Autodesk Inventor part; units mm, degrees
(part 3 of 15)
  line L366 (-4.016, 12.192) -> (-4.016, 13.208)
  arc A1008 (-3.9652, 13.208) -> (-4.0668, 13.208) centre (-4.016, 13.208) ccw
  arc A1009 (-4.0668, 12.192) -> (-3.9652, 12.192) centre (-4.016, 12.192) ccw
  arc A1010 (39.084, 48.5588) -> (39.084, 48.4572) centre (39.084, 48.508) ccw
  line L367 (-17.016, 17.208) -> (-14.984, 17.208)
  arc A1011 (-14.984, 17.1572) -> (-14.984, 17.2588) centre (-14.984, 17.208) ccw
  arc A1012 (-17.016, 17.2588) -> (-17.016, 17.1572) centre (-17.016, 17.208) ccw
  line L368 (-14.984, 17.208) -> (-14.984, 16.192)
  arc A1013 (-15.0348, 16.192) -> (-14.9332, 16.192) centre (-14.984, 16.192) ccw
  arc A1014 (-14.9332, 17.208) -> (-15.0348, 17.208) centre (-14.984, 17.208) ccw
  line L369 (-14.984, 16.192) -> (-17.016, 16.192)
  arc A1015 (-17.016, 16.2428) -> (-17.016, 16.1412) centre (-17.016, 16.192) ccw
  arc A1016 (-14.984, 16.1412) -> (-14.984, 16.2428) centre (-14.984, 16.192) ccw
  line L370 (-17.016, 16.192) -> (-17.016, 17.208)
  arc A1017 (-16.9652, 17.208) -> (-17.0668, 17.208) centre (-17.016, 17.208) ccw
  arc A1018 (-17.0668, 16.192) -> (-16.9652, 16.192) centre (-17.016, 16.192) ccw
  line L371 (41.116, 48.508) -> (41.116, 47.492)
  line L372 (-16.984, 0.192) -> (-19.016, 0.192)
  arc A1019 (-19.016, 0.2428) -> (-19.016, 0.1412) centre (-19.016, 0.192) ccw
  arc A1020 (-16.984, 0.1412) -> (-16.984, 0.2428) centre (-16.984, 0.192) ccw
  line L373 (-19.016, 0.192) -> (-19.016, 1.208)
  arc A1021 (-18.9652, 1.208) -> (-19.0668, 1.208) centre (-19.016, 1.208) ccw
  arc A1022 (-19.0668, 0.192) -> (-18.9652, 0.192) centre (-19.016, 0.192) ccw
  line L374 (-19.016, 1.208) -> (-16.984, 1.208)
  arc A1023 (-16.984, 1.1572) -> (-16.984, 1.2588) centre (-16.984, 1.208) ccw
  arc A1024 (-19.016, 1.2588) -> (-19.016, 1.1572) centre (-19.016, 1.208) ccw
  line L375 (-16.984, 1.208) -> (-16.984, 0.192)
  arc A1025 (-17.0348, 0.192) -> (-16.9332, 0.192) centre (-16.984, 0.192) ccw
  arc A1026 (-16.9332, 1.208) -> (-17.0348, 1.208) centre (-16.984, 1.208) ccw
  arc A1027 (41.0652, 47.492) -> (41.1668, 47.492) centre (41.116, 47.492) ccw
  line L376 (7.008, 13.216) -> (7.008, 11.184)
  arc A1028 (6.9572, 11.184) -> (7.0588, 11.184) centre (7.008, 11.184) ccw
  arc A1029 (7.0588, 13.216) -> (6.9572, 13.216) centre (7.008, 13.216) ccw
  line L377 (7.008, 11.184) -> (5.992, 11.184)
  arc A1030 (5.992, 11.2348) -> (5.992, 11.1332) centre (5.992, 11.184) ccw
  arc A1031 (7.008, 11.1332) -> (7.008, 11.2348) centre (7.008, 11.184) ccw
  line L378 (5.992, 11.184) -> (5.992, 13.216)
  arc A1032 (6.0428, 13.216) -> (5.9412, 13.216) centre (5.992, 13.216) ccw
  arc A1033 (5.9412, 11.184) -> (6.0428, 11.184) centre (5.992, 11.184) ccw
  line L379 (5.992, 13.216) -> (7.008, 13.216)
  arc A1034 (7.008, 13.1652) -> (7.008, 13.2668) centre (7.008, 13.216) ccw
  arc A1035 (5.992, 13.2668) -> (5.992, 13.1652) centre (5.992, 13.216) ccw
  arc A1036 (41.1668, 48.508) -> (41.0652, 48.508) centre (41.116, 48.508) ccw
  line L380 (-15.984, 6.192) -> (-18.016, 6.192)
  arc A1037 (-18.016, 6.2428) -> (-18.016, 6.1412) centre (-18.016, 6.192) ccw
  arc A1038 (-15.984, 6.1412) -> (-15.984, 6.2428) centre (-15.984, 6.192) ccw
  line L381 (-18.016, 6.192) -> (-18.016, 7.208)
  arc A1039 (-17.9652, 7.208) -> (-18.0668, 7.208) centre (-18.016, 7.208) ccw
  arc A1040 (-18.0668, 6.192) -> (-17.9652, 6.192) centre (-18.016, 6.192) ccw
  line L382 (-18.016, 7.208) -> (-15.984, 7.208)
  arc A1041 (-15.984, 7.1572) -> (-15.984, 7.2588) centre (-15.984, 7.208) ccw
  arc A1042 (-18.016, 7.2588) -> (-18.016, 7.1572) centre (-18.016, 7.208) ccw
  line L383 (-15.984, 7.208) -> (-15.984, 6.192)
  arc A1043 (-16.0348, 6.192) -> (-15.9332, 6.192) centre (-15.984, 6.192) ccw
  arc A1044 (-15.9332, 7.208) -> (-16.0348, 7.208) centre (-15.984, 7.208) ccw
  line L384 (41.116, 48.492) -> (39.084, 48.492)
  line L385 (-1.984, 11.192) -> (-4.016, 11.192)
  arc A1045 (-4.016, 11.2428) -> (-4.016, 11.1412) centre (-4.016, 11.192) ccw
  arc A1046 (-1.984, 11.1412) -> (-1.984, 11.2428) centre (-1.984, 11.192) ccw
  line L386 (-4.016, 11.192) -> (-4.016, 12.208)
  arc A1047 (-3.9652, 12.208) -> (-4.0668, 12.208) centre (-4.016, 12.208) ccw
  arc A1048 (-4.0668, 11.192) -> (-3.9652, 11.192) centre (-4.016, 11.192) ccw
  line L387 (-4.016, 12.208) -> (-1.984, 12.208)
  arc A1049 (-1.984, 12.1572) -> (-1.984, 12.2588) centre (-1.984, 12.208) ccw
  arc A1050 (-4.016, 12.2588) -> (-4.016, 12.1572) centre (-4.016, 12.208) ccw
  line L388 (-1.984, 12.208) -> (-1.984, 11.192)
  arc A1051 (-2.0348, 11.192) -> (-1.9332, 11.192) centre (-1.984, 11.192) ccw
  arc A1052 (-1.9332, 12.208) -> (-2.0348, 12.208) centre (-1.984, 12.208) ccw
  arc A1053 (39.084, 48.5428) -> (39.084, 48.4412) centre (39.084, 48.492) ccw
  line L389 (-17.984, 17.192) -> (-20.016, 17.192)
  arc A1054 (-20.016, 17.2428) -> (-20.016, 17.1412) centre (-20.016, 17.192) ccw
  arc A1055 (-17.984, 17.1412) -> (-17.984, 17.2428) centre (-17.984, 17.192) ccw
  line L390 (-20.016, 17.192) -> (-20.016, 18.208)
  arc A1056 (-19.9652, 18.208) -> (-20.0668, 18.208) centre (-20.016, 18.208) ccw
  arc A1057 (-20.0668, 17.192) -> (-19.9652, 17.192) centre (-20.016, 17.192) ccw
  line L391 (-20.016, 18.208) -> (-17.984, 18.208)
  arc A1058 (-17.984, 18.1572) -> (-17.984, 18.2588) centre (-17.984, 18.208) ccw
  arc A1059 (-20.016, 18.2588) -> (-20.016, 18.1572) centre (-20.016, 18.208) ccw
  line L392 (-17.984, 18.208) -> (-17.984, 17.192)
  arc A1060 (-18.0348, 17.192) -> (-17.9332, 17.192) centre (-17.984, 17.192) ccw
  arc A1061 (-17.9332, 18.208) -> (-18.0348, 18.208) centre (-17.984, 18.208) ccw
  arc A1062 (41.116, 48.4412) -> (41.116, 48.5428) centre (41.116, 48.492) ccw
  line L393 (-18.008, 12.184) -> (-18.008, 14.216)
  arc A1063 (-17.9572, 14.216) -> (-18.0588, 14.216) centre (-18.008, 14.216) ccw
  arc A1064 (-18.0588, 12.184) -> (-17.9572, 12.184) centre (-18.008, 12.184) ccw
  line L394 (-18.008, 14.216) -> (-16.992, 14.216)
  arc A1065 (-16.992, 14.1652) -> (-16.992, 14.2668) centre (-16.992, 14.216) ccw
  arc A1066 (-18.008, 14.2668) -> (-18.008, 14.1652) centre (-18.008, 14.216) ccw
  line L395 (-16.992, 14.216) -> (-16.992, 12.184)
  arc A1067 (-17.0428, 12.184) -> (-16.9412, 12.184) centre (-16.992, 12.184) ccw
  arc A1068 (-16.9412, 14.216) -> (-17.0428, 14.216) centre (-16.992, 14.216) ccw
  line L396 (-16.992, 12.184) -> (-18.008, 12.184)
  arc A1069 (-18.008, 12.2348) -> (-18.008, 12.1332) centre (-18.008, 12.184) ccw
  arc A1070 (-16.992, 12.1332) -> (-16.992, 12.2348) centre (-16.992, 12.184) ccw
  line L397 (39.084, 48.492) -> (39.084, 49.508)
  line L398 (-14.992, 10.216) -> (-14.992, 8.184)
  arc A1071 (-15.0428, 8.184) -> (-14.9412, 8.184) centre (-14.992, 8.184) ccw
  arc A1072 (-14.9412, 10.216) -> (-15.0428, 10.216) centre (-14.992, 10.216) ccw
  line L399 (-14.992, 8.184) -> (-16.008, 8.184)
  arc A1073 (-16.008, 8.2348) -> (-16.008, 8.1332) centre (-16.008, 8.184) ccw
  arc A1074 (-14.992, 8.1332) -> (-14.992, 8.2348) centre (-14.992, 8.184) ccw
  line L400 (-16.008, 8.184) -> (-16.008, 10.216)
  arc A1075 (-15.9572, 10.216) -> (-16.0588, 10.216) centre (-16.008, 10.216) ccw
  arc A1076 (-16.0588, 8.184) -> (-15.9572, 8.184) centre (-16.008, 8.184) ccw
  line L401 (-16.008, 10.216) -> (-14.992, 10.216)
  arc A1077 (-14.992, 10.1652) -> (-14.992, 10.2668) centre (-14.992, 10.216) ccw
  arc A1078 (-16.008, 10.2668) -> (-16.008, 10.1652) centre (-16.008, 10.216) ccw
  arc A1079 (39.1348, 49.508) -> (39.0332, 49.508) centre (39.084, 49.508) ccw
  line L402 (3.103, 14.835) -> (5.897, 14.835)
  arc A1080 (5.897, 14.7842) -> (5.897, 14.8858) centre (5.897, 14.835) ccw
  arc A1081 (3.103, 14.8858) -> (3.103, 14.7842) centre (3.103, 14.835) ccw
  line L403 (5.897, 14.835) -> (5.897, 13.565)
  arc A1082 (5.8462, 13.565) -> (5.9478, 13.565) centre (5.897, 13.565) ccw
  arc A1083 (5.9478, 14.835) -> (5.8462, 14.835) centre (5.897, 14.835) ccw
  line L404 (5.897, 13.565) -> (3.103, 13.565)
  arc A1084 (3.103, 13.6158) -> (3.103, 13.5142) centre (3.103, 13.565) ccw
  arc A1085 (5.897, 13.5142) -> (5.897, 13.6158) centre (5.897, 13.565) ccw
  line L405 (3.103, 13.565) -> (3.103, 14.835)
  arc A1086 (3.1538, 14.835) -> (3.0522, 14.835) centre (3.103, 14.835) ccw
  arc A1087 (3.0522, 13.565) -> (3.1538, 13.565) centre (3.103, 13.565) ccw
  arc A1088 (39.0332, 48.492) -> (39.1348, 48.492) centre (39.084, 48.492) ccw
  line L406 (-3.008, 7.184) -> (-3.008, 9.216)
  arc A1089 (-2.9572, 9.216) -> (-3.0588, 9.216) centre (-3.008, 9.216) ccw
  arc A1090 (-3.0588, 7.184) -> (-2.9572, 7.184) centre (-3.008, 7.184) ccw
  line L407 (-3.008, 9.216) -> (-1.992, 9.216)
  arc A1091 (-1.992, 9.1652) -> (-1.992, 9.2668) centre (-1.992, 9.216) ccw
  arc A1092 (-3.008, 9.2668) -> (-3.008, 9.1652) centre (-3.008, 9.216) ccw
  line L408 (-1.992, 9.216) -> (-1.992, 7.184)
  arc A1093 (-2.0428, 7.184) -> (-1.9412, 7.184) centre (-1.992, 7.184) ccw
  arc A1094 (-1.9412, 9.216) -> (-2.0428, 9.216) centre (-1.992, 9.216) ccw
  line L409 (-1.992, 7.184) -> (-3.008, 7.184)
  arc A1095 (-3.008, 7.2348) -> (-3.008, 7.1332) centre (-3.008, 7.184) ccw
  arc A1096 (-1.992, 7.1332) -> (-1.992, 7.2348) centre (-1.992, 7.184) ccw
  line L410 (39.084, 49.508) -> (41.116, 49.508)
  line L411 (-15.984, 4.192) -> (-18.016, 4.192)
  arc A1097 (-18.016, 4.2428) -> (-18.016, 4.1412) centre (-18.016, 4.192) ccw
  arc A1098 (-15.984, 4.1412) -> (-15.984, 4.2428) centre (-15.984, 4.192) ccw
  line L412 (-18.016, 4.192) -> (-18.016, 5.208)
  arc A1099 (-17.9652, 5.208) -> (-18.0668, 5.208) centre (-18.016, 5.208) ccw
  arc A1100 (-18.0668, 4.192) -> (-17.9652, 4.192) centre (-18.016, 4.192) ccw
  line L413 (-18.016, 5.208) -> (-15.984, 5.208)
  arc A1101 (-15.984, 5.1572) -> (-15.984, 5.2588) centre (-15.984, 5.208) ccw
  arc A1102 (-18.016, 5.2588) -> (-18.016, 5.1572) centre (-18.016, 5.208) ccw
  line L414 (-15.984, 5.208) -> (-15.984, 4.192)
  arc A1103 (-16.0348, 4.192) -> (-15.9332, 4.192) centre (-15.984, 4.192) ccw
  arc A1104 (-15.9332, 5.208) -> (-16.0348, 5.208) centre (-15.984, 5.208) ccw
  arc A1105 (41.116, 49.4572) -> (41.116, 49.5588) centre (41.116, 49.508) ccw
  line L415 (-12.397, 4.835) -> (-9.603, 4.835)
  arc A1106 (-9.603, 4.7842) -> (-9.603, 4.8858) centre (-9.603, 4.835) ccw
  arc A1107 (-12.397, 4.8858) -> (-12.397, 4.7842) centre (-12.397, 4.835) ccw
  line L416 (-9.603, 4.835) -> (-9.603, 3.565)
  arc A1108 (-9.6538, 3.565) -> (-9.5522, 3.565) centre (-9.603, 3.565) ccw
  arc A1109 (-9.5522, 4.835) -> (-9.6538, 4.835) centre (-9.603, 4.835) ccw
  line L417 (-9.603, 3.565) -> (-12.397, 3.565)
  arc A1110 (-12.397, 3.6158) -> (-12.397, 3.5142) centre (-12.397, 3.565) ccw
  arc A1111 (-9.603, 3.5142) -> (-9.603, 3.6158) centre (-9.603, 3.565) ccw
  line L418 (-12.397, 3.565) -> (-12.397, 4.835)
  arc A1112 (-12.3462, 4.835) -> (-12.4478, 4.835) centre (-12.397, 4.835) ccw
  arc A1113 (-12.4478, 3.565) -> (-12.3462, 3.565) centre (-12.397, 3.565) ccw
  arc A1114 (39.084, 49.5588) -> (39.084, 49.4572) centre (39.084, 49.508) ccw
  line L419 (-6.165, 16.097) -> (-6.165, 13.303)
  arc A1115 (-6.2158, 13.303) -> (-6.1142, 13.303) centre (-6.165, 13.303) ccw
  arc A1116 (-6.1142, 16.097) -> (-6.2158, 16.097) centre (-6.165, 16.097) ccw
  line L420 (-6.165, 13.303) -> (-7.435, 13.303)
  arc A1117 (-7.435, 13.3538) -> (-7.435, 13.2522) centre (-7.435, 13.303) ccw
  arc A1118 (-6.165, 13.2522) -> (-6.165, 13.3538) centre (-6.165, 13.303) ccw
  line L421 (-7.435, 13.303) -> (-7.435, 16.097)
  arc A1119 (-7.3842, 16.097) -> (-7.4858, 16.097) centre (-7.435, 16.097) ccw
  arc A1120 (-7.4858, 13.303) -> (-7.3842, 13.303) centre (-7.435, 13.303) ccw
  line L422 (-7.435, 16.097) -> (-6.165, 16.097)
  arc A1121 (-6.165, 16.0462) -> (-6.165, 16.1478) centre (-6.165, 16.097) ccw
  arc A1122 (-7.435, 16.1478) -> (-7.435, 16.0462) centre (-7.435, 16.097) ccw
  line L423 (41.116, 49.508) -> (41.116, 48.492)
  line L424 (-5.984, 12.192) -> (-8.016, 12.192)
  arc A1123 (-8.016, 12.2428) -> (-8.016, 12.1412) centre (-8.016, 12.192) ccw
  arc A1124 (-5.984, 12.1412) -> (-5.984, 12.2428) centre (-5.984, 12.192) ccw
  line L425 (-8.016, 12.192) -> (-8.016, 13.208)
  arc A1125 (-7.9652, 13.208) -> (-8.0668, 13.208) centre (-8.016, 13.208) ccw
  arc A1126 (-8.0668, 12.192) -> (-7.9652, 12.192) centre (-8.016, 12.192) ccw
  line L426 (-8.016, 13.208) -> (-5.984, 13.208)
  arc A1127 (-5.984, 13.1572) -> (-5.984, 13.2588) centre (-5.984, 13.208) ccw
  arc A1128 (-8.016, 13.2588) -> (-8.016, 13.1572) centre (-8.016, 13.208) ccw
  line L427 (-5.984, 13.208) -> (-5.984, 12.192)
  arc A1129 (-6.0348, 12.192) -> (-5.9332, 12.192) centre (-5.984, 12.192) ccw
  arc A1130 (-5.9332, 13.208) -> (-6.0348, 13.208) centre (-5.984, 13.208) ccw
  arc A1131 (41.0652, 48.492) -> (41.1668, 48.492) centre (41.116, 48.492) ccw
  line L428 (-9.865, 12.097) -> (-9.865, 9.303)
  arc A1132 (-9.9158, 9.303) -> (-9.8142, 9.303) centre (-9.865, 9.303) ccw
  arc A1133 (-9.8142, 12.097) -> (-9.9158, 12.097) centre (-9.865, 12.097) ccw
  line L429 (-9.865, 9.303) -> (-11.135, 9.303)
  arc A1134 (-11.135, 9.3538) -> (-11.135, 9.2522) centre (-11.135, 9.303) ccw
  arc A1135 (-9.865, 9.2522) -> (-9.865, 9.3538) centre (-9.865, 9.303) ccw
  line L430 (-11.135, 9.303) -> (-11.135, 12.097)
  arc A1136 (-11.0842, 12.097) -> (-11.1858, 12.097) centre (-11.135, 12.097) ccw
  arc A1137 (-11.1858, 9.303) -> (-11.0842, 9.303) centre (-11.135, 9.303) ccw
  line L431 (-11.135, 12.097) -> (-9.865, 12.097)
  arc A1138 (-9.865, 12.0462) -> (-9.865, 12.1478) centre (-9.865, 12.097) ccw
  arc A1139 (-11.135, 12.1478) -> (-11.135, 12.0462) centre (-11.135, 12.097) ccw
  arc A1140 (41.1668, 49.508) -> (41.0652, 49.508) centre (41.116, 49.508) ccw
  line L432 (-7.565, 16.097) -> (-7.565, 13.303)
  arc A1141 (-7.6158, 13.303) -> (-7.5142, 13.303) centre (-7.565, 13.303) ccw
  arc A1142 (-7.5142, 16.097) -> (-7.6158, 16.097) centre (-7.565, 16.097) ccw
  line L433 (-7.565, 13.303) -> (-8.835, 13.303)
  arc A1143 (-8.835, 13.3538) -> (-8.835, 13.2522) centre (-8.835, 13.303) ccw
  arc A1144 (-7.565, 13.2522) -> (-7.565, 13.3538) centre (-7.565, 13.303) ccw
  line L434 (-8.835, 13.303) -> (-8.835, 16.097)
  arc A1145 (-8.7842, 16.097) -> (-8.8858, 16.097) centre (-8.835, 16.097) ccw
  arc A1146 (-8.8858, 13.303) -> (-8.7842, 13.303) centre (-8.835, 13.303) ccw
  line L435 (-8.835, 16.097) -> (-7.565, 16.097)
  arc A1147 (-7.565, 16.0462) -> (-7.565, 16.1478) centre (-7.565, 16.097) ccw
  arc A1148 (-8.835, 16.1478) -> (-8.835, 16.0462) centre (-8.835, 16.097) ccw
  line L436 (41.116, 49.492) -> (39.084, 49.492)
  line L437 (-16.187, 8.076) -> (-21.013, 8.076)
  arc A1149 (-21.013, 8.1268) -> (-21.013, 8.0252) centre (-21.013, 8.076) ccw
  arc A1150 (-16.187, 8.0252) -> (-16.187, 8.1268) centre (-16.187, 8.076) ccw
  line L438 (-21.013, 8.076) -> (-21.013, 11.124)
  arc A1151 (-20.9622, 11.124) -> (-21.0638, 11.124) centre (-21.013, 11.124) ccw
  arc A1152 (-21.0638, 8.076) -> (-20.9622, 8.076) centre (-21.013, 8.076) ccw
  line L439 (-21.013, 11.124) -> (-16.187, 11.124)
  arc A1153 (-16.187, 11.0732) -> (-16.187, 11.1748) centre (-16.187, 11.124) ccw
  arc A1154 (-21.013, 11.1748) -> (-21.013, 11.0732) centre (-21.013, 11.124) ccw
  line L440 (-16.187, 11.124) -> (-16.187, 8.076)
  arc A1155 (-16.2378, 8.076) -> (-16.1362, 8.076) centre (-16.187, 8.076) ccw
  arc A1156 (-16.1362, 11.124) -> (-16.2378, 11.124) centre (-16.187, 11.124) ccw
  arc A1157 (39.084, 49.5428) -> (39.084, 49.4412) centre (39.084, 49.492) ccw
  line L441 (-24.8542, 11.089) -> (-21.1458, 11.089)
  arc A1158 (-21.1458, 11.0382) -> (-21.1458, 11.1398) centre (-21.1458, 11.089) ccw
  arc A1159 (-24.8542, 11.1398) -> (-24.8542, 11.0382) centre (-24.8542, 11.089) ccw
  line L442 (-21.1458, 11.089) -> (-21.1458, 9.311)
  arc A1160 (-21.1966, 9.311) -> (-21.095, 9.311) centre (-21.1458, 9.311) ccw
  arc A1161 (-21.095, 11.089) -> (-21.1966, 11.089) centre (-21.1458, 11.089) ccw
  line L443 (-21.1458, 9.311) -> (-24.8542, 9.311)
  arc A1162 (-24.8542, 9.3618) -> (-24.8542, 9.2602) centre (-24.8542, 9.311) ccw
  arc A1163 (-21.1458, 9.2602) -> (-21.1458, 9.3618) centre (-21.1458, 9.311) ccw
  line L444 (-24.8542, 9.311) -> (-24.8542, 11.089)
  arc A1164 (-24.8034, 11.089) -> (-24.905, 11.089) centre (-24.8542, 11.089) ccw
  arc A1165 (-24.905, 9.311) -> (-24.8034, 9.311) centre (-24.8542, 9.311) ccw
  arc A1166 (41.116, 49.4412) -> (41.116, 49.5428) centre (41.116, 49.492) ccw
  line L445 (-4.016, -2.792) -> (-1.984, -2.792)
  arc A1167 (-1.984, -2.8428) -> (-1.984, -2.7412) centre (-1.984, -2.792) ccw
  arc A1168 (-4.016, -2.7412) -> (-4.016, -2.8428) centre (-4.016, -2.792) ccw
  line L446 (-1.984, -2.792) -> (-1.984, -3.808)
  arc A1169 (-2.0348, -3.808) -> (-1.9332, -3.808) centre (-1.984, -3.808) ccw
  arc A1170 (-1.9332, -2.792) -> (-2.0348, -2.792) centre (-1.984, -2.792) ccw
  line L447 (-1.984, -3.808) -> (-4.016, -3.808)
  arc A1171 (-4.016, -3.7572) -> (-4.016, -3.8588) centre (-4.016, -3.808) ccw
  arc A1172 (-1.984, -3.8588) -> (-1.984, -3.7572) centre (-1.984, -3.808) ccw
  line L448 (-4.016, -3.808) -> (-4.016, -2.792)
  arc A1173 (-3.9652, -2.792) -> (-4.0668, -2.792) centre (-4.016, -2.792) ccw
  arc A1174 (-4.0668, -3.808) -> (-3.9652, -3.808) centre (-4.016, -3.808) ccw
  line L449 (39.084, 49.492) -> (39.084, 50.508)
  line L450 (-3.635, -7.697) -> (-3.635, -4.903)
  arc A1175 (-3.5842, -4.903) -> (-3.6858, -4.903) centre (-3.635, -4.903) ccw
  arc A1176 (-3.6858, -7.697) -> (-3.5842, -7.697) centre (-3.635, -7.697) ccw
  line L451 (-3.635, -4.903) -> (-2.365, -4.903)
  arc A1177 (-2.365, -4.9538) -> (-2.365, -4.8522) centre (-2.365, -4.903) ccw
  arc A1178 (-3.635, -4.8522) -> (-3.635, -4.9538) centre (-3.635, -4.903) ccw
  line L452 (-2.365, -4.903) -> (-2.365, -7.697)
  arc A1179 (-2.4158, -7.697) -> (-2.3142, -7.697) centre (-2.365, -7.697) ccw
  arc A1180 (-2.3142, -4.903) -> (-2.4158, -4.903) centre (-2.365, -4.903) ccw
  line L453 (-2.365, -7.697) -> (-3.635, -7.697)
  arc A1181 (-3.635, -7.6462) -> (-3.635, -7.7478) centre (-3.635, -7.697) ccw
  arc A1182 (-2.365, -7.7478) -> (-2.365, -7.6462) centre (-2.365, -7.697) ccw
  arc A1183 (39.1348, 50.508) -> (39.0332, 50.508) centre (39.084, 50.508) ccw
  line L454 (-13.811, 21.0542) -> (-13.811, 17.3458)
  arc A1184 (-13.8618, 17.3458) -> (-13.7602, 17.3458) centre (-13.811, 17.3458) ccw
  arc A1185 (-13.7602, 21.0542) -> (-13.8618, 21.0542) centre (-13.811, 21.0542) ccw
  line L455 (-13.811, 17.3458) -> (-15.589, 17.3458)
  arc A1186 (-15.589, 17.3966) -> (-15.589, 17.295) centre (-15.589, 17.3458) ccw
  arc A1187 (-13.811, 17.295) -> (-13.811, 17.3966) centre (-13.811, 17.3458) ccw
  line L456 (-15.589, 17.3458) -> (-15.589, 21.0542)
  arc A1188 (-15.5382, 21.0542) -> (-15.6398, 21.0542) centre (-15.589, 21.0542) ccw
  arc A1189 (-15.6398, 17.3458) -> (-15.5382, 17.3458) centre (-15.589, 17.3458) ccw
  line L457 (-15.589, 21.0542) -> (-13.811, 21.0542)
  arc A1190 (-13.811, 21.0034) -> (-13.811, 21.105) centre (-13.811, 21.0542) ccw
  arc A1191 (-15.589, 21.105) -> (-15.589, 21.0034) centre (-15.589, 21.0542) ccw
  arc A1192 (39.0332, 49.492) -> (39.1348, 49.492) centre (39.084, 49.492) ccw
  line L458 (-4.016, -1.792) -> (-1.984, -1.792)
  arc A1193 (-1.984, -1.8428) -> (-1.984, -1.7412) centre (-1.984, -1.792) ccw
  arc A1194 (-4.016, -1.7412) -> (-4.016, -1.8428) centre (-4.016, -1.792) ccw
  line L459 (-1.984, -1.792) -> (-1.984, -2.808)
  arc A1195 (-2.0348, -2.808) -> (-1.9332, -2.808) centre (-1.984, -2.808) ccw
  arc A1196 (-1.9332, -1.792) -> (-2.0348, -1.792) centre (-1.984, -1.792) ccw
  line L460 (-1.984, -2.808) -> (-4.016, -2.808)
  arc A1197 (-4.016, -2.7572) -> (-4.016, -2.8588) centre (-4.016, -2.808) ccw
  arc A1198 (-1.984, -2.8588) -> (-1.984, -2.7572) centre (-1.984, -2.808) ccw
  line L461 (-4.016, -2.808) -> (-4.016, -1.792)
  arc A1199 (-3.9652, -1.792) -> (-4.0668, -1.792) centre (-4.016, -1.792) ccw
  arc A1200 (-4.0668, -2.808) -> (-3.9652, -2.808) centre (-4.016, -2.808) ccw
  line L462 (39.084, 50.508) -> (41.116, 50.508)
  line L463 (1.016, -1.808) -> (-1.016, -1.808)
  arc A1201 (-1.016, -1.7572) -> (-1.016, -1.8588) centre (-1.016, -1.808) ccw
  arc A1202 (1.016, -1.8588) -> (1.016, -1.7572) centre (1.016, -1.808) ccw
  line L464 (-1.016, -1.808) -> (-1.016, -0.792)
  arc A1203 (-0.9652, -0.792) -> (-1.0668, -0.792) centre (-1.016, -0.792) ccw
  arc A1204 (-1.0668, -1.808) -> (-0.9652, -1.808) centre (-1.016, -1.808) ccw
  line L465 (-1.016, -0.792) -> (1.016, -0.792)
  arc A1205 (1.016, -0.8428) -> (1.016, -0.7412) centre (1.016, -0.792) ccw
  arc A1206 (-1.016, -0.7412) -> (-1.016, -0.8428) centre (-1.016, -0.792) ccw
  line L466 (1.016, -0.792) -> (1.016, -1.808)
  arc A1207 (0.9652, -1.808) -> (1.0668, -1.808) centre (1.016, -1.808) ccw
  arc A1208 (1.0668, -0.792) -> (0.9652, -0.792) centre (1.016, -0.792) ccw
  arc A1209 (41.116, 50.4572) -> (41.116, 50.5588) centre (41.116, 50.508) ccw
  line L467 (-15.611, 21.0542) -> (-15.611, 17.3458)
  arc A1210 (-15.6618, 17.3458) -> (-15.5602, 17.3458) centre (-15.611, 17.3458) ccw
  arc A1211 (-15.5602, 21.0542) -> (-15.6618, 21.0542) centre (-15.611, 21.0542) ccw
  line L468 (-15.611, 17.3458) -> (-17.389, 17.3458)
  arc A1212 (-17.389, 17.3966) -> (-17.389, 17.295) centre (-17.389, 17.3458) ccw
  arc A1213 (-15.611, 17.295) -> (-15.611, 17.3966) centre (-15.611, 17.3458) ccw
  line L469 (-17.389, 17.3458) -> (-17.389, 21.0542)
  arc A1214 (-17.3382, 21.0542) -> (-17.4398, 21.0542) centre (-17.389, 21.0542) ccw
  arc A1215 (-17.4398, 17.3458) -> (-17.3382, 17.3458) centre (-17.389, 17.3458) ccw
  line L470 (-17.389, 21.0542) -> (-15.611, 21.0542)
  arc A1216 (-15.611, 21.0034) -> (-15.611, 21.105) centre (-15.611, 21.0542) ccw
  arc A1217 (-17.389, 21.105) -> (-17.389, 21.0034) centre (-17.389, 21.0542) ccw
  arc A1218 (39.084, 50.5588) -> (39.084, 50.4572) centre (39.084, 50.508) ccw
  line L471 (-21.1458, -10.789) -> (-24.8542, -10.789)
  arc A1219 (-24.8542, -10.7382) -> (-24.8542, -10.8398) centre (-24.8542, -10.789) ccw
  arc A1220 (-21.1458, -10.8398) -> (-21.1458, -10.7382) centre (-21.1458, -10.789) ccw
  line L472 (-24.8542, -10.789) -> (-24.8542, -9.011)
  arc A1221 (-24.8034, -9.011) -> (-24.905, -9.011) centre (-24.8542, -9.011) ccw
  arc A1222 (-24.905, -10.789) -> (-24.8034, -10.789) centre (-24.8542, -10.789) ccw
  line L473 (-24.8542, -9.011) -> (-21.1458, -9.011)
  arc A1223 (-21.1458, -9.0618) -> (-21.1458, -8.9602) centre (-21.1458, -9.011) ccw
  arc A1224 (-24.8542, -8.9602) -> (-24.8542, -9.0618) centre (-24.8542, -9.011) ccw
  line L474 (-21.1458, -9.011) -> (-21.1458, -10.789)
  arc A1225 (-21.1966, -10.789) -> (-21.095, -10.789) centre (-21.1458, -10.789) ccw
  arc A1226 (-21.095, -9.011) -> (-21.1966, -9.011) centre (-21.1458, -9.011) ccw
  line L475 (41.116, 50.508) -> (41.116, 49.492)
  line L476 (0.992, -4.816) -> (0.992, -2.784)
  arc A1227 (1.0428, -2.784) -> (0.9412, -2.784) centre (0.992, -2.784) ccw
  arc A1228 (0.9412, -4.816) -> (1.0428, -4.816) centre (0.992, -4.816) ccw
  line L477 (0.992, -2.784) -> (2.008, -2.784)
  arc A1229 (2.008, -2.8348) -> (2.008, -2.7332) centre (2.008, -2.784) ccw
  arc A1230 (0.992, -2.7332) -> (0.992, -2.8348) centre (0.992, -2.784) ccw
  line L478 (2.008, -2.784) -> (2.008, -4.816)
  arc A1231 (1.9572, -4.816) -> (2.0588, -4.816) centre (2.008, -4.816) ccw
  arc A1232 (2.0588, -2.784) -> (1.9572, -2.784) centre (2.008, -2.784) ccw
  line L479 (2.008, -4.816) -> (0.992, -4.816)
  arc A1233 (0.992, -4.7652) -> (0.992, -4.8668) centre (0.992, -4.816) ccw
  arc A1234 (2.008, -4.8668) -> (2.008, -4.7652) centre (2.008, -4.816) ccw
  arc A1235 (41.0652, 49.492) -> (41.1668, 49.492) centre (41.116, 49.492) ccw
  line L480 (-6.016, -1.792) -> (-3.984, -1.792)
  arc A1236 (-3.984, -1.8428) -> (-3.984, -1.7412) centre (-3.984, -1.792) ccw
  arc A1237 (-6.016, -1.7412) -> (-6.016, -1.8428) centre (-6.016, -1.792) ccw
  line L481 (-3.984, -1.792) -> (-3.984, -2.808)
  arc A1238 (-4.0348, -2.808) -> (-3.9332, -2.808) centre (-3.984, -2.808) ccw
  arc A1239 (-3.9332, -1.792) -> (-4.0348, -1.792) centre (-3.984, -1.792) ccw
  line L482 (-3.984, -2.808) -> (-6.016, -2.808)
  arc A1240 (-6.016, -2.7572) -> (-6.016, -2.8588) centre (-6.016, -2.808) ccw
  arc A1241 (-3.984, -2.8588) -> (-3.984, -2.7572) centre (-3.984, -2.808) ccw
  line L483 (-6.016, -2.808) -> (-6.016, -1.792)
  arc A1242 (-5.9652, -1.792) -> (-6.0668, -1.792) centre (-6.016, -1.792) ccw
  arc A1243 (-6.0668, -2.808) -> (-5.9652, -2.808) centre (-6.016, -2.808) ccw
  arc A1244 (41.1668, 50.508) -> (41.0652, 50.508) centre (41.116, 50.508) ccw
  line L484 (0.008, -2.784) -> (0.008, -4.816)
  arc A1245 (-0.0428, -4.816) -> (0.0588, -4.816) centre (0.008, -4.816) ccw
  arc A1246 (0.0588, -2.784) -> (-0.0428, -2.784) centre (0.008, -2.784) ccw
  line L485 (0.008, -4.816) -> (-1.008, -4.816)
  arc A1247 (-1.008, -4.7652) -> (-1.008, -4.8668) centre (-1.008, -4.816) ccw
  arc A1248 (0.008, -4.8668) -> (0.008, -4.7652) centre (0.008, -4.816) ccw
  line L486 (-1.008, -4.816) -> (-1.008, -2.784)
  arc A1249 (-0.9572, -2.784) -> (-1.0588, -2.784) centre (-1.008, -2.784) ccw
  arc A1250 (-1.0588, -4.816) -> (-0.9572, -4.816) centre (-1.008, -4.816) ccw
  line L487 (-1.008, -2.784) -> (0.008, -2.784)
  arc A1251 (0.008, -2.8348) -> (0.008, -2.7332) centre (0.008, -2.784) ccw
  arc A1252 (-1.008, -2.7332) -> (-1.008, -2.8348) centre (-1.008, -2.784) ccw
  line L488 (41.116, 50.492) -> (39.084, 50.492)
  line L489 (-12.011, 21.0542) -> (-12.011, 17.3458)
  arc A1253 (-12.0618, 17.3458) -> (-11.9602, 17.3458) centre (-12.011, 17.3458) ccw
  arc A1254 (-11.9602, 21.0542) -> (-12.0618, 21.0542) centre (-12.011, 21.0542) ccw
  line L490 (-12.011, 17.3458) -> (-13.789, 17.3458)
  arc A1255 (-13.789, 17.3966) -> (-13.789, 17.295) centre (-13.789, 17.3458) ccw
  arc A1256 (-12.011, 17.295) -> (-12.011, 17.3966) centre (-12.011, 17.3458) ccw
  line L491 (-13.789, 17.3458) -> (-13.789, 21.0542)
  arc A1257 (-13.7382, 21.0542) -> (-13.8398, 21.0542) centre (-13.789, 21.0542) ccw
  arc A1258 (-13.8398, 17.3458) -> (-13.7382, 17.3458) centre (-13.789, 17.3458) ccw
  line L492 (-13.789, 21.0542) -> (-12.011, 21.0542)
  arc A1259 (-12.011, 21.0034) -> (-12.011, 21.105) centre (-12.011, 21.0542) ccw
  arc A1260 (-13.789, 21.105) -> (-13.789, 21.0034) centre (-13.789, 21.0542) ccw
  arc A1261 (39.084, 50.5428) -> (39.084, 50.4412) centre (39.084, 50.492) ccw
  line L493 (-0.992, -1.784) -> (-0.992, -3.816)
  arc A1262 (-1.0428, -3.816) -> (-0.9412, -3.816) centre (-0.992, -3.816) ccw
  arc A1263 (-0.9412, -1.784) -> (-1.0428, -1.784) centre (-0.992, -1.784) ccw
  line L494 (-0.992, -3.816) -> (-2.008, -3.816)
  arc A1264 (-2.008, -3.7652) -> (-2.008, -3.8668) centre (-2.008, -3.816) ccw
  arc A1265 (-0.992, -3.8668) -> (-0.992, -3.7652) centre (-0.992, -3.816) ccw
  line L495 (-2.008, -3.816) -> (-2.008, -1.784)
  arc A1266 (-1.9572, -1.784) -> (-2.0588, -1.784) centre (-2.008, -1.784) ccw
  arc A1267 (-2.0588, -3.816) -> (-1.9572, -3.816) centre (-2.008, -3.816) ccw
  line L496 (-2.008, -1.784) -> (-0.992, -1.784)
  arc A1268 (-0.992, -1.8348) -> (-0.992, -1.7332) centre (-0.992, -1.784) ccw
  arc A1269 (-2.008, -1.7332) -> (-2.008, -1.8348) centre (-2.008, -1.784) ccw
  arc A1270 (41.116, 50.4412) -> (41.116, 50.5428) centre (41.116, 50.492) ccw
  line L497 (2.008, 1.216) -> (2.008, -0.816)
  arc A1271 (1.9572, -0.816) -> (2.0588, -0.816) centre (2.008, -0.816) ccw
  arc A1272 (2.0588, 1.216) -> (1.9572, 1.216) centre (2.008, 1.216) ccw
  line L498 (2.008, -0.816) -> (0.992, -0.816)
  arc A1273 (0.992, -0.7652) -> (0.992, -0.8668) centre (0.992, -0.816) ccw
  arc A1274 (2.008, -0.8668) -> (2.008, -0.7652) centre (2.008, -0.816) ccw
  line L499 (0.992, -0.816) -> (0.992, 1.216)
  arc A1275 (1.0428, 1.216) -> (0.9412, 1.216) centre (0.992, 1.216) ccw
  arc A1276 (0.9412, -0.816) -> (1.0428, -0.816) centre (0.992, -0.816) ccw
  line L500 (0.992, 1.216) -> (2.008, 1.216)
  arc A1277 (2.008, 1.1652) -> (2.008, 1.2668) centre (2.008, 1.216) ccw
  arc A1278 (0.992, 1.2668) -> (0.992, 1.1652) centre (0.992, 1.216) ccw
  line L501 (39.084, 50.492) -> (39.084, 51.508)
  line L502 (-0.984, -0.808) -> (-3.016, -0.808)
  arc A1279 (-3.016, -0.7572) -> (-3.016, -0.8588) centre (-3.016, -0.808) ccw
  arc A1280 (-0.984, -0.8588) -> (-0.984, -0.7572) centre (-0.984, -0.808) ccw
  line L503 (-3.016, -0.808) -> (-3.016, 0.208)
  arc A1281 (-2.9652, 0.208) -> (-3.0668, 0.208) centre (-3.016, 0.208) ccw
  arc A1282 (-3.0668, -0.808) -> (-2.9652, -0.808) centre (-3.016, -0.808) ccw
  line L504 (-3.016, 0.208) -> (-0.984, 0.208)
  arc A1283 (-0.984, 0.1572) -> (-0.984, 0.2588) centre (-0.984, 0.208) ccw
  arc A1284 (-3.016, 0.2588) -> (-3.016, 0.1572) centre (-3.016, 0.208) ccw
  line L505 (-0.984, 0.208) -> (-0.984, -0.808)
  arc A1285 (-1.0348, -0.808) -> (-0.9332, -0.808) centre (-0.984, -0.808) ccw
  arc A1286 (-0.9332, 0.208) -> (-1.0348, 0.208) centre (-0.984, 0.208) ccw
  arc A1287 (39.1348, 51.508) -> (39.0332, 51.508) centre (39.084, 51.508) ccw
  line L506 (-2.984, -10.808) -> (-5.016, -10.808)
  arc A1288 (-5.016, -10.7572) -> (-5.016, -10.8588) centre (-5.016, -10.808) ccw
  arc A1289 (-2.984, -10.8588) -> (-2.984, -10.7572) centre (-2.984, -10.808) ccw
  line L507 (-5.016, -10.808) -> (-5.016, -9.792)
  arc A1290 (-4.9652, -9.792) -> (-5.0668, -9.792) centre (-5.016, -9.792) ccw
  arc A1291 (-5.0668, -10.808) -> (-4.9652, -10.808) centre (-5.016, -10.808) ccw
  line L508 (-5.016, -9.792) -> (-2.984, -9.792)
  arc A1292 (-2.984, -9.8428) -> (-2.984, -9.7412) centre (-2.984, -9.792) ccw
  arc A1293 (-5.016, -9.7412) -> (-5.016, -9.8428) centre (-5.016, -9.792) ccw
  line L509 (-2.984, -9.792) -> (-2.984, -10.808)
  arc A1294 (-3.0348, -10.808) -> (-2.9332, -10.808) centre (-2.984, -10.808) ccw
  arc A1295 (-2.9332, -9.792) -> (-3.0348, -9.792) centre (-2.984, -9.792) ccw
  arc A1296 (39.0332, 50.492) -> (39.1348, 50.492) centre (39.084, 50.492) ccw
  line L510 (-7.008, -1.816) -> (-7.008, 0.216)
  arc A1297 (-6.9572, 0.216) -> (-7.0588, 0.216) centre (-7.008, 0.216) ccw
  arc A1298 (-7.0588, -1.816) -> (-6.9572, -1.816) centre (-7.008, -1.816) ccw
  line L511 (-7.008, 0.216) -> (-5.992, 0.216)
  arc A1299 (-5.992, 0.1652) -> (-5.992, 0.2668) centre (-5.992, 0.216) ccw
  arc A1300 (-7.008, 0.2668) -> (-7.008, 0.1652) centre (-7.008, 0.216) ccw
  line L512 (-5.992, 0.216) -> (-5.992, -1.816)
  arc A1301 (-6.0428, -1.816) -> (-5.9412, -1.816) centre (-5.992, -1.816) ccw
  arc A1302 (-5.9412, 0.216) -> (-6.0428, 0.216) centre (-5.992, 0.216) ccw
  line L513 (-5.992, -1.816) -> (-7.008, -1.816)
  arc A1303 (-7.008, -1.7652) -> (-7.008, -1.8668) centre (-7.008, -1.816) ccw
  arc A1304 (-5.992, -1.8668) -> (-5.992, -1.7652) centre (-5.992, -1.816) ccw
  line L514 (39.084, 51.508) -> (41.116, 51.508)
  line L515 (-3.984, -6.808) -> (-6.016, -6.808)
  arc A1305 (-6.016, -6.7572) -> (-6.016, -6.8588) centre (-6.016, -6.808) ccw
  arc A1306 (-3.984, -6.8588) -> (-3.984, -6.7572) centre (-3.984, -6.808) ccw
  line L516 (-6.016, -6.808) -> (-6.016, -5.792)
  arc A1307 (-5.9652, -5.792) -> (-6.0668, -5.792) centre (-6.016, -5.792) ccw
  arc A1308 (-6.0668, -6.808) -> (-5.9652, -6.808) centre (-6.016, -6.808) ccw
  line L517 (-6.016, -5.792) -> (-3.984, -5.792)
  arc A1309 (-3.984, -5.8428) -> (-3.984, -5.7412) centre (-3.984, -5.792) ccw
  arc A1310 (-6.016, -5.7412) -> (-6.016, -5.8428) centre (-6.016, -5.792) ccw
  line L518 (-3.984, -5.792) -> (-3.984, -6.808)
  arc A1311 (-4.0348, -6.808) -> (-3.9332, -6.808) centre (-3.984, -6.808) ccw
  arc A1312 (-3.9332, -5.792) -> (-4.0348, -5.792) centre (-3.984, -5.792) ccw
  arc A1313 (41.116, 51.4572) -> (41.116, 51.5588) centre (41.116, 51.508) ccw
  line L519 (-24.8542, 2.089) -> (-21.1458, 2.089)
  arc A1314 (-21.1458, 2.0382) -> (-21.1458, 2.1398) centre (-21.1458, 2.089) ccw
  arc A1315 (-24.8542, 2.1398) -> (-24.8542, 2.0382) centre (-24.8542, 2.089) ccw
  line L520 (-21.1458, 2.089) -> (-21.1458, 0.311)
  arc A1316 (-21.1966, 0.311) -> (-21.095, 0.311) centre (-21.1458, 0.311) ccw
  arc A1317 (-21.095, 2.089) -> (-21.1966, 2.089) centre (-21.1458, 2.089) ccw
  line L521 (-21.1458, 0.311) -> (-24.8542, 0.311)
  arc A1318 (-24.8542, 0.3618) -> (-24.8542, 0.2602) centre (-24.8542, 0.311) ccw
  arc A1319 (-21.1458, 0.2602) -> (-21.1458, 0.3618) centre (-21.1458, 0.311) ccw
  line L522 (-24.8542, 0.311) -> (-24.8542, 2.089)
  arc A1320 (-24.8034, 2.089) -> (-24.905, 2.089) centre (-24.8542, 2.089) ccw
  arc A1321 (-24.905, 0.311) -> (-24.8034, 0.311) centre (-24.8542, 0.311) ccw
  arc A1322 (39.084, 51.5588) -> (39.084, 51.4572) centre (39.084, 51.508) ccw
  line L523 (-18.992, 0.216) -> (-18.992, -1.816)
  arc A1323 (-19.0428, -1.816) -> (-18.9412, -1.816) centre (-18.992, -1.816) ccw
  arc A1324 (-18.9412, 0.216) -> (-19.0428, 0.216) centre (-18.992, 0.216) ccw
  line L524 (-18.992, -1.816) -> (-20.008, -1.816)
  arc A1325 (-20.008, -1.7652) -> (-20.008, -1.8668) centre (-20.008, -1.816) ccw
  arc A1326 (-18.992, -1.8668) -> (-18.992, -1.7652) centre (-18.992, -1.816) ccw
  line L525 (-20.008, -1.816) -> (-20.008, 0.216)
  arc A1327 (-19.9572, 0.216) -> (-20.0588, 0.216) centre (-20.008, 0.216) ccw
  arc A1328 (-20.0588, -1.816) -> (-19.9572, -1.816) centre (-20.008, -1.816) ccw
  line L526 (-20.008, 0.216) -> (-18.992, 0.216)
  arc A1329 (-18.992, 0.1652) -> (-18.992, 0.2668) centre (-18.992, 0.216) ccw
  arc A1330 (-20.008, 0.2668) -> (-20.008, 0.1652) centre (-20.008, 0.216) ccw
  line L527 (41.116, 51.508) -> (41.116, 50.492)
  line L528 (6.008, -4.784) -> (6.008, -6.816)
  arc A1331 (5.9572, -6.816) -> (6.0588, -6.816) centre (6.008, -6.816) ccw
  arc A1332 (6.0588, -4.784) -> (5.9572, -4.784) centre (6.008, -4.784) ccw
  line L529 (6.008, -6.816) -> (4.992, -6.816)
  arc A1333 (4.992, -6.7652) -> (4.992, -6.8668) centre (4.992, -6.816) ccw
  arc A1334 (6.008, -6.8668) -> (6.008, -6.7652) centre (6.008, -6.816) ccw
  line L530 (4.992, -6.816) -> (4.992, -4.784)
  arc A1335 (5.0428, -4.784) -> (4.9412, -4.784) centre (4.992, -4.784) ccw
  arc A1336 (4.9412, -6.816) -> (5.0428, -6.816) centre (4.992, -6.816) ccw
  line L531 (4.992, -4.784) -> (6.008, -4.784)
  arc A1337 (6.008, -4.8348) -> (6.008, -4.7332) centre (6.008, -4.784) ccw
  arc A1338 (4.992, -4.7332) -> (4.992, -4.8348) centre (4.992, -4.784) ccw
  arc A1339 (41.0652, 50.492) -> (41.1668, 50.492) centre (41.116, 50.492) ccw
  line L532 (-24.8542, 7.489) -> (-21.1458, 7.489)
  arc A1340 (-21.1458, 7.4382) -> (-21.1458, 7.5398) centre (-21.1458, 7.489) ccw
  arc A1341 (-24.8542, 7.5398) -> (-24.8542, 7.4382) centre (-24.8542, 7.489) ccw
  line L533 (-21.1458, 7.489) -> (-21.1458, 5.711)
  arc A1342 (-21.1966, 5.711) -> (-21.095, 5.711) centre (-21.1458, 5.711) ccw
  arc A1343 (-21.095, 7.489) -> (-21.1966, 7.489) centre (-21.1458, 7.489) ccw
  line L534 (-21.1458, 5.711) -> (-24.8542, 5.711)
  arc A1344 (-24.8542, 5.7618) -> (-24.8542, 5.6602) centre (-24.8542, 5.711) ccw
  arc A1345 (-21.1458, 5.6602) -> (-21.1458, 5.7618) centre (-21.1458, 5.711) ccw
  line L535 (-24.8542, 5.711) -> (-24.8542, 7.489)
  arc A1346 (-24.8034, 7.489) -> (-24.905, 7.489) centre (-24.8542, 7.489) ccw
  arc A1347 (-24.905, 5.711) -> (-24.8034, 5.711) centre (-24.8542, 5.711) ccw
  arc A1348 (41.1668, 51.508) -> (41.0652, 51.508) centre (41.116, 51.508) ccw
  line L536 (20.711, -24.6542) -> (20.711, -20.9458)
  arc A1349 (20.7618, -20.9458) -> (20.6602, -20.9458) centre (20.711, -20.9458) ccw
  arc A1350 (20.6602, -24.6542) -> (20.7618, -24.6542) centre (20.711, -24.6542) ccw
  line L537 (20.711, -20.9458) -> (22.489, -20.9458)
  arc A1351 (22.489, -20.9966) -> (22.489, -20.895) centre (22.489, -20.9458) ccw
  arc A1352 (20.711, -20.895) -> (20.711, -20.9966) centre (20.711, -20.9458) ccw
  line L538 (22.489, -20.9458) -> (22.489, -24.6542)
  arc A1353 (22.4382, -24.6542) -> (22.5398, -24.6542) centre (22.489, -24.6542) ccw
  arc A1354 (22.5398, -20.9458) -> (22.4382, -20.9458) centre (22.489, -20.9458) ccw
  line L539 (22.489, -24.6542) -> (20.711, -24.6542)
  arc A1355 (20.711, -24.6034) -> (20.711, -24.705) centre (20.711, -24.6542) ccw
  arc A1356 (22.489, -24.705) -> (22.489, -24.6034) centre (22.489, -24.6542) ccw
  line L540 (41.116, 44.992) -> (39.084, 44.992)
  line L541 (22.511, -24.6542) -> (22.511, -20.9458)
  arc A1357 (22.5618, -20.9458) -> (22.4602, -20.9458) centre (22.511, -20.9458) ccw
  arc A1358 (22.4602, -24.6542) -> (22.5618, -24.6542) centre (22.511, -24.6542) ccw
  line L542 (22.511, -20.9458) -> (24.289, -20.9458)
  arc A1359 (24.289, -20.9966) -> (24.289, -20.895) centre (24.289, -20.9458) ccw
  arc A1360 (22.511, -20.895) -> (22.511, -20.9966) centre (22.511, -20.9458) ccw
  line L543 (24.289, -20.9458) -> (24.289, -24.6542)
  arc A1361 (24.2382, -24.6542) -> (24.3398, -24.6542) centre (24.289, -24.6542) ccw
  arc A1362 (24.3398, -20.9458) -> (24.2382, -20.9458) centre (24.289, -20.9458) ccw
  line L544 (24.289, -24.6542) -> (22.511, -24.6542)
  arc A1363 (22.511, -24.6034) -> (22.511, -24.705) centre (22.511, -24.6542) ccw
  arc A1364 (24.289, -24.705) -> (24.289, -24.6034) centre (24.289, -24.6542) ccw
  arc A1365 (39.084, 45.0428) -> (39.084, 44.9412) centre (39.084, 44.992) ccw
  line L545 (-9.984, -0.808) -> (-12.016, -0.808)
  arc A1366 (-12.016, -0.7572) -> (-12.016, -0.8588) centre (-12.016, -0.808) ccw
  arc A1367 (-9.984, -0.8588) -> (-9.984, -0.7572) centre (-9.984, -0.808) ccw
  line L546 (-12.016, -0.808) -> (-12.016, 0.208)
  arc A1368 (-11.9652, 0.208) -> (-12.0668, 0.208) centre (-12.016, 0.208) ccw
  arc A1369 (-12.0668, -0.808) -> (-11.9652, -0.808) centre (-12.016, -0.808) ccw
  line L547 (-12.016, 0.208) -> (-9.984, 0.208)
  arc A1370 (-9.984, 0.1572) -> (-9.984, 0.2588) centre (-9.984, 0.208) ccw
  arc A1371 (-12.016, 0.2588) -> (-12.016, 0.1572) centre (-12.016, 0.208) ccw
  line L548 (-9.984, 0.208) -> (-9.984, -0.808)
  arc A1372 (-10.0348, -0.808) -> (-9.9332, -0.808) centre (-9.984, -0.808) ccw
  arc A1373 (-9.9332, 0.208) -> (-10.0348, 0.208) centre (-9.984, 0.208) ccw
  arc A1374 (41.116, 44.9412) -> (41.116, 45.0428) centre (41.116, 44.992) ccw
  line L549 (-24.8542, 9.289) -> (-21.1458, 9.289)
  arc A1375 (-21.1458, 9.2382) -> (-21.1458, 9.3398) centre (-21.1458, 9.289) ccw
  arc A1376 (-24.8542, 9.3398) -> (-24.8542, 9.2382) centre (-24.8542, 9.289) ccw
  line L550 (-21.1458, 9.289) -> (-21.1458, 7.511)
  arc A1377 (-21.1966, 7.511) -> (-21.095, 7.511) centre (-21.1458, 7.511) ccw
  arc A1378 (-21.095, 9.289) -> (-21.1966, 9.289) centre (-21.1458, 9.289) ccw
  line L551 (-21.1458, 7.511) -> (-24.8542, 7.511)
  arc A1379 (-24.8542, 7.5618) -> (-24.8542, 7.4602) centre (-24.8542, 7.511) ccw
  arc A1380 (-21.1458, 7.4602) -> (-21.1458, 7.5618) centre (-21.1458, 7.511) ccw
  line L552 (-24.8542, 7.511) -> (-24.8542, 9.289)
  arc A1381 (-24.8034, 9.289) -> (-24.905, 9.289) centre (-24.8542, 9.289) ccw
  arc A1382 (-24.905, 7.511) -> (-24.8034, 7.511) centre (-24.8542, 7.511) ccw
  line L553 (39.084, 44.992) -> (39.084, 46.008)
  line L554 (3.016, 5.192) -> (0.984, 5.192)
  arc A1383 (0.984, 5.2428) -> (0.984, 5.1412) centre (0.984, 5.192) ccw
  arc A1384 (3.016, 5.1412) -> (3.016, 5.2428) centre (3.016, 5.192) ccw
  line L555 (0.984, 5.192) -> (0.984, 6.208)
  arc A1385 (1.0348, 6.208) -> (0.9332, 6.208) centre (0.984, 6.208) ccw
  arc A1386 (0.9332, 5.192) -> (1.0348, 5.192) centre (0.984, 5.192) ccw
  line L556 (0.984, 6.208) -> (3.016, 6.208)
  arc A1387 (3.016, 6.1572) -> (3.016, 6.2588) centre (3.016, 6.208) ccw
  arc A1388 (0.984, 6.2588) -> (0.984, 6.1572) centre (0.984, 6.208) ccw
  line L557 (3.016, 6.208) -> (3.016, 5.192)
  arc A1389 (2.9652, 5.192) -> (3.0668, 5.192) centre (3.016, 5.192) ccw
  arc A1390 (3.0668, 6.208) -> (2.9652, 6.208) centre (3.016, 6.208) ccw
  arc A1391 (39.1348, 46.008) -> (39.0332, 46.008) centre (39.084, 46.008) ccw
  line L558 (-24.8542, 3.889) -> (-21.1458, 3.889)
  arc A1392 (-21.1458, 3.8382) -> (-21.1458, 3.9398) centre (-21.1458, 3.889) ccw
  arc A1393 (-24.8542, 3.9398) -> (-24.8542, 3.8382) centre (-24.8542, 3.889) ccw
  line L559 (-21.1458, 3.889) -> (-21.1458, 2.111)
  arc A1394 (-21.1966, 2.111) -> (-21.095, 2.111) centre (-21.1458, 2.111) ccw
  arc A1395 (-21.095, 3.889) -> (-21.1966, 3.889) centre (-21.1458, 3.889) ccw
  line L560 (-21.1458, 2.111) -> (-24.8542, 2.111)
  arc A1396 (-24.8542, 2.1618) -> (-24.8542, 2.0602) centre (-24.8542, 2.111) ccw
  arc A1397 (-21.1458, 2.0602) -> (-21.1458, 2.1618) centre (-21.1458, 2.111) ccw
  line L561 (-24.8542, 2.111) -> (-24.8542, 3.889)
  arc A1398 (-24.8034, 3.889) -> (-24.905, 3.889) centre (-24.8542, 3.889) ccw
  arc A1399 (-24.905, 2.111) -> (-24.8034, 2.111) centre (-24.8542, 2.111) ccw
  arc A1400 (39.0332, 44.992) -> (39.1348, 44.992) centre (39.084, 44.992) ccw
  line L562 (-24.8542, 5.689) -> (-21.1458, 5.689)
  arc A1401 (-21.1458, 5.6382) -> (-21.1458, 5.7398) centre (-21.1458, 5.689) ccw
  arc A1402 (-24.8542, 5.7398) -> (-24.8542, 5.6382) centre (-24.8542, 5.689) ccw
  line L563 (-21.1458, 5.689) -> (-21.1458, 3.911)
  arc A1403 (-21.1966, 3.911) -> (-21.095, 3.911) centre (-21.1458, 3.911) ccw
  arc A1404 (-21.095, 5.689) -> (-21.1966, 5.689) centre (-21.1458, 5.689) ccw
  line L564 (-21.1458, 3.911) -> (-24.8542, 3.911)
  arc A1405 (-24.8542, 3.9618) -> (-24.8542, 3.8602) centre (-24.8542, 3.911) ccw
  arc A1406 (-21.1458, 3.8602) -> (-21.1458, 3.9618) centre (-21.1458, 3.911) ccw
  line L565 (-24.8542, 3.911) -> (-24.8542, 5.689)
  arc A1407 (-24.8034, 5.689) -> (-24.905, 5.689) centre (-24.8542, 5.689) ccw
  arc A1408 (-24.905, 3.911) -> (-24.8034, 3.911) centre (-24.8542, 3.911) ccw
  line L566 (39.084, 46.008) -> (41.116, 46.008)
  line L567 (-24.8542, 0.289) -> (-21.1458, 0.289)
  arc A1409 (-21.1458, 0.2382) -> (-21.1458, 0.3398) centre (-21.1458, 0.289) ccw
  arc A1410 (-24.8542, 0.3398) -> (-24.8542, 0.2382) centre (-24.8542, 0.289) ccw
  line L568 (-21.1458, 0.289) -> (-21.1458, -1.489)
  arc A1411 (-21.1966, -1.489) -> (-21.095, -1.489) centre (-21.1458, -1.489) ccw
  arc A1412 (-21.095, 0.289) -> (-21.1966, 0.289) centre (-21.1458, 0.289) ccw
  line L569 (-21.1458, -1.489) -> (-24.8542, -1.489)
  arc A1413 (-24.8542, -1.4382) -> (-24.8542, -1.5398) centre (-24.8542, -1.489) ccw
  arc A1414 (-21.1458, -1.5398) -> (-21.1458, -1.4382) centre (-21.1458, -1.489) ccw
  line L570 (-24.8542, -1.489) -> (-24.8542, 0.289)
  arc A1415 (-24.8034, 0.289) -> (-24.905, 0.289) centre (-24.8542, 0.289) ccw
  arc A1416 (-24.905, -1.489) -> (-24.8034, -1.489) centre (-24.8542, -1.489) ccw
  arc A1417 (41.116, 45.9572) -> (41.116, 46.0588) centre (41.116, 46.008) ccw
  line L571 (-5.016, 0.208) -> (-2.984, 0.208)
  arc A1418 (-2.984, 0.1572) -> (-2.984, 0.2588) centre (-2.984, 0.208) ccw
  arc A1419 (-5.016, 0.2588) -> (-5.016, 0.1572) centre (-5.016, 0.208) ccw
  line L572 (-2.984, 0.208) -> (-2.984, -0.808)
  arc A1420 (-3.0348, -0.808) -> (-2.9332, -0.808) centre (-2.984, -0.808) ccw
  arc A1421 (-2.9332, 0.208) -> (-3.0348, 0.208) centre (-2.984, 0.208) ccw
  line L573 (-2.984, -0.808) -> (-5.016, -0.808)
  arc A1422 (-5.016, -0.7572) -> (-5.016, -0.8588) centre (-5.016, -0.808) ccw
  arc A1423 (-2.984, -0.8588) -> (-2.984, -0.7572) centre (-2.984, -0.808) ccw
  line L574 (-5.016, -0.808) -> (-5.016, 0.208)
  arc A1424 (-4.9652, 0.208) -> (-5.0668, 0.208) centre (-5.016, 0.208) ccw
  arc A1425 (-5.0668, -0.808) -> (-4.9652, -0.808) centre (-5.016, -0.808) ccw
  arc A1426 (39.084, 46.0588) -> (39.084, 45.9572) centre (39.084, 46.008) ccw
  line L575 (-5.008, 0.184) -> (-5.008, 2.216)
  arc A1427 (-4.9572, 2.216) -> (-5.0588, 2.216) centre (-5.008, 2.216) ccw
  arc A1428 (-5.0588, 0.184) -> (-4.9572, 0.184) centre (-5.008, 0.184) ccw
  line L576 (-5.008, 2.216) -> (-3.992, 2.216)
  arc A1429 (-3.992, 2.1652) -> (-3.992, 2.2668) centre (-3.992, 2.216) ccw
  arc A1430 (-5.008, 2.2668) -> (-5.008, 2.1652) centre (-5.008, 2.216) ccw
  line L577 (-3.992, 2.216) -> (-3.992, 0.184)
  arc A1431 (-4.0428, 0.184) -> (-3.9412, 0.184) centre (-3.992, 0.184) ccw
  arc A1432 (-3.9412, 2.216) -> (-4.0428, 2.216) centre (-3.992, 2.216) ccw
  line L578 (-3.992, 0.184) -> (-5.008, 0.184)
  arc A1433 (-5.008, 0.2348) -> (-5.008, 0.1332) centre (-5.008, 0.184) ccw
  arc A1434 (-3.992, 0.1332) -> (-3.992, 0.2348) centre (-3.992, 0.184) ccw
  line L579 (41.116, 46.008) -> (41.116, 44.992)
  line L580 (-16.992, 3.216) -> (-16.992, 1.184)
  arc A1435 (-17.0428, 1.184) -> (-16.9412, 1.184) centre (-16.992, 1.184) ccw
  arc A1436 (-16.9412, 3.216) -> (-17.0428, 3.216) centre (-16.992, 3.216) ccw
  line L581 (-16.992, 1.184) -> (-18.008, 1.184)
  arc A1437 (-18.008, 1.2348) -> (-18.008, 1.1332) centre (-18.008, 1.184) ccw
  arc A1438 (-16.992, 1.1332) -> (-16.992, 1.2348) centre (-16.992, 1.184) ccw
  line L582 (-18.008, 1.184) -> (-18.008, 3.216)
  arc A1439 (-17.9572, 3.216) -> (-18.0588, 3.216) centre (-18.008, 3.216) ccw
  arc A1440 (-18.0588, 1.184) -> (-17.9572, 1.184) centre (-18.008, 1.184) ccw
  line L583 (-18.008, 3.216) -> (-16.992, 3.216)
  arc A1441 (-16.992, 3.1652) -> (-16.992, 3.2668) centre (-16.992, 3.216) ccw
  arc A1442 (-18.008, 3.2668) -> (-18.008, 3.1652) centre (-18.008, 3.216) ccw
  arc A1443 (41.0652, 44.992) -> (41.1668, 44.992) centre (41.116, 44.992) ccw
  line L584 (-22.184, -23.408) -> (-24.216, -23.408)
  arc A1444 (-24.216, -23.3572) -> (-24.216, -23.4588) centre (-24.216, -23.408) ccw
  arc A1445 (-22.184, -23.4588) -> (-22.184, -23.3572) centre (-22.184, -23.408) ccw
  line L585 (-24.216, -23.408) -> (-24.216, -22.392)
  arc A1446 (-24.1652, -22.392) -> (-24.2668, -22.392) centre (-24.216, -22.392) ccw
  arc A1447 (-24.2668, -23.408) -> (-24.1652, -23.408) centre (-24.216, -23.408) ccw
  line L586 (-24.216, -22.392) -> (-22.184, -22.392)
  arc A1448 (-22.184, -22.4428) -> (-22.184, -22.3412) centre (-22.184, -22.392) ccw
  arc A1449 (-24.216, -22.3412) -> (-24.216, -22.4428) centre (-24.216, -22.392) ccw
  line L587 (-22.184, -22.392) -> (-22.184, -23.408)
  arc A1450 (-22.2348, -23.408) -> (-22.1332, -23.408) centre (-22.184, -23.408) ccw
  arc A1451 (-22.1332, -22.392) -> (-22.2348, -22.392) centre (-22.184, -22.392) ccw
  arc A1452 (41.1668, 46.008) -> (41.0652, 46.008) centre (41.116, 46.008) ccw
  line L588 (20.916, 20.192) -> (18.884, 20.192)
  arc A1453 (18.884, 20.2428) -> (18.884, 20.1412) centre (18.884, 20.192) ccw
  arc A1454 (20.916, 20.1412) -> (20.916, 20.2428) centre (20.916, 20.192) ccw
  line L589 (18.884, 20.192) -> (18.884, 21.208)
  arc A1455 (18.9348, 21.208) -> (18.8332, 21.208) centre (18.884, 21.208) ccw
  arc A1456 (18.8332, 20.192) -> (18.9348, 20.192) centre (18.884, 20.192) ccw
  line L590 (18.884, 21.208) -> (20.916, 21.208)
  arc A1457 (20.916, 21.1572) -> (20.916, 21.2588) centre (20.916, 21.208) ccw
  arc A1458 (18.884, 21.2588) -> (18.884, 21.1572) centre (18.884, 21.208) ccw
  line L591 (20.916, 21.208) -> (20.916, 20.192)
  arc A1459 (20.8652, 20.192) -> (20.9668, 20.192) centre (20.916, 20.192) ccw
  arc A1460 (20.9668, 21.208) -> (20.8652, 21.208) centre (20.916, 21.208) ccw
  line L592 (41.116, 43.992) -> (39.084, 43.992)
  line L593 (16.684, 21.208) -> (18.716, 21.208)
  arc A1461 (18.716, 21.1572) -> (18.716, 21.2588) centre (18.716, 21.208) ccw
  arc A1462 (16.684, 21.2588) -> (16.684, 21.1572) centre (16.684, 21.208) ccw
  line L594 (18.716, 21.208) -> (18.716, 20.192)
  arc A1463 (18.6652, 20.192) -> (18.7668, 20.192) centre (18.716, 20.192) ccw
  arc A1464 (18.7668, 21.208) -> (18.6652, 21.208) centre (18.716, 21.208) ccw
  line L595 (18.716, 20.192) -> (16.684, 20.192)
  arc A1465 (16.684, 20.2428) -> (16.684, 20.1412) centre (16.684, 20.192) ccw
  arc A1466 (18.716, 20.1412) -> (18.716, 20.2428) centre (18.716, 20.192) ccw
  line L596 (16.684, 20.192) -> (16.684, 21.208)
  arc A1467 (16.7348, 21.208) -> (16.6332, 21.208) centre (16.684, 21.208) ccw
  arc A1468 (16.6332, 20.192) -> (16.7348, 20.192) centre (16.684, 20.192) ccw
  arc A1469 (39.084, 44.0428) -> (39.084, 43.9412) centre (39.084, 43.992) ccw
  line L597 (22.884, 17.208) -> (24.916, 17.208)
  arc A1470 (24.916, 17.1572) -> (24.916, 17.2588) centre (24.916, 17.208) ccw
  arc A1471 (22.884, 17.2588) -> (22.884, 17.1572) centre (22.884, 17.208) ccw
  line L598 (24.916, 17.208) -> (24.916, 16.192)
  arc A1472 (24.8652, 16.192) -> (24.9668, 16.192) centre (24.916, 16.192) ccw
  arc A1473 (24.9668, 17.208) -> (24.8652, 17.208) centre (24.916, 17.208) ccw
  line L599 (24.916, 16.192) -> (22.884, 16.192)
  arc A1474 (22.884, 16.2428) -> (22.884, 16.1412) centre (22.884, 16.192) ccw
  arc A1475 (24.916, 16.1412) -> (24.916, 16.2428) centre (24.916, 16.192) ccw
  line L600 (22.884, 16.192) -> (22.884, 17.208)
  arc A1476 (22.9348, 17.208) -> (22.8332, 17.208) centre (22.884, 17.208) ccw
  arc A1477 (22.8332, 16.192) -> (22.9348, 16.192) centre (22.884, 16.192) ccw
  arc A1478 (41.116, 43.9412) -> (41.116, 44.0428) centre (41.116, 43.992) ccw
  line L601 (20.916, 9.792) -> (18.884, 9.792)
  arc A1479 (18.884, 9.8428) -> (18.884, 9.7412) centre (18.884, 9.792) ccw
  arc A1480 (20.916, 9.7412) -> (20.916, 9.8428) centre (20.916, 9.792) ccw
  line L602 (18.884, 9.792) -> (18.884, 10.808)
  arc A1481 (18.9348, 10.808) -> (18.8332, 10.808) centre (18.884, 10.808) ccw
  arc A1482 (18.8332, 9.792) -> (18.9348, 9.792) centre (18.884, 9.792) ccw
  line L603 (18.884, 10.808) -> (20.916, 10.808)
  arc A1483 (20.916, 10.7572) -> (20.916, 10.8588) centre (20.916, 10.808) ccw
  arc A1484 (18.884, 10.8588) -> (18.884, 10.7572) centre (18.884, 10.808) ccw
  line L604 (20.916, 10.808) -> (20.916, 9.792)
  arc A1485 (20.8652, 9.792) -> (20.9668, 9.792) centre (20.916, 9.792) ccw
  arc A1486 (20.9668, 10.808) -> (20.8652, 10.808) centre (20.916, 10.808) ccw
  line L605 (39.084, 43.992) -> (39.084, 45.008)